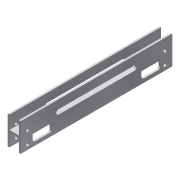
# Autodesk Inventor part: car frame
Saved by Autodesk Inventor 2015 (Build 190159000, 159)
## iProperties
Created: 2014-07-18
Part Number: car frame
Material: Generic
Document SubType Name: Modeling
Designer: Owner
Density: 1 g/cm^3
Appearance: Aluminum - Polished
Author: Owner
Autodesk Inventor part; units mm, degrees
ref_plane "YZ Plane" through (0, 0, 0) normal (1, 0, 0) x (0, 1, 0)
ref_plane "XZ Plane" through (0, 0, 0) normal (0, 1, 0) x (-1, 0, 0)
ref_plane "XY Plane" through (0, 0, 0) normal (0, 0, 1) x (1, 0, 0)
sketch "Sketch1" plane through (0, 0, 0) normal (0, 0, 1) x (1, 0, 0)
  line L0 (-6.35, 0) -> (6.35, 0)
  line L1 (-6.35, -2.3876) -> (6.35, -2.3876)
  line L2 (6.35, 0) -> (6.35, 17.8562)
  line L3 (6.35, 17.8562) -> (8.7376, 17.8562)
  line L4 (8.7376, 17.8562) -> (8.7376, -20.2438)
  line L5 (8.7376, -20.2438) -> (6.35, -20.2438)
  line L6 (6.35, -20.2438) -> (6.35, -2.3876)
  line L7 (-6.35, -2.3876) -> (-6.35, -20.2438)
  line L8 (-6.35, -20.2438) -> (-8.7376, -20.2438)
  line L9 (-8.7376, -20.2438) -> (-8.7376, 17.8562)
  line L10 (-8.7376, 17.8562) -> (-6.35, 17.8562)
  line L11 (-6.35, 17.8562) -> (-6.35, 0)
  point P0 (0, 0)
  point P1 (0, 0)
  dimension "d9" = 12.7
  dimension "d10" = 2.3876
  dimension "d11" = 17.8562
  dimension "d12" = 38.1
  dimension "d13" = 2.3876
  dimension "d14" = 2.3876
  dimension "d15" = 2.3876
  dimension "d16" = 17.8562
  dimension "d17" = 17.8562
  constraints: 24 end point, 7 parallel, 3 perpendicular, 2 collinear, 1 coincident, 1 horizontal, 1 midpoint
  measures "d9" distance of L0.start L0.end
  measures "d10" distance between parallel lines of L1 L0
  measures "d11" distance of L0.end L2.end
  measures "d12" distance of L3.end L4.end
  measures "d13" distance of L2.end L3.end
  measures "d14" distance of L4.end L5.end
  measures "d15" distance of L7.end L8.end
  measures "d16" distance of L10.end L0.start
  measures "d17" distance of L1.start L7.end
extrude "Extrusion1" add sketch "Sketch1" against normal blind 203.2
sketch "Sketch2" plane through (8.7376, -20.2438, 0) normal (1, 0, 0) x (0, 0, -1)
  point P0 (0, 0)
  point P1 (9.525, 6.35)
  dimension "d20" = 9.525
  dimension "d21" = 6.35
  measures "d20" horizontal distance of point (9.525, 6.35) point (0, 0)
  measures "d21" vertical distance of point (0, 0) point (9.525, 6.35)
hole "Hole1" at (8.7376, -13.8938, -9.525) direction (-1, 0, 0) diameter 4.2164 end through all
sketch "Sketch3" plane through (8.7376, -20.2438, 0) normal (1, 0, 0) x (0, 0, -1)
  point P0 (0, 38.1)
  point P1 (9.525, 23.0188)
  dimension "d29" = 15.0813
  dimension "d30" = 9.525
  measures "d29" vertical distance of point (0, 38.1) point (9.525, 23.019)
  measures "d30" horizontal distance of point (0, 38.1) point (9.525, 23.019)
hole "Hole2" at (8.7376, 2.775, -9.525) direction (-1, 0, 0) diameter 4.2164 end through all
sketch "Sketch4" plane through (8.7376, -20.2438, 0) normal (1, 0, 0) x (0, 0, -1)
  circle A0 centre (9.525, 23.0188) radius 2.1082 projected
  circle A1 centre (9.525, 6.35) radius 2.1082 projected
  line L0 (0, 0) -> (203.2, 0) projected
  line L1 (0, 38.1) -> (203.2, 38.1) projected
  line L2 (101.6, 38.1) -> (101.6, 0) construction
  circle A2 centre (193.675, 23.0188) radius 2.1082
  circle A3 centre (193.675, 6.35) radius 2.1082
  constraints: 2 centre point, 2 end point, 2 midpoint, 2 symmetric about line, 2 other
hole "Hole3" at (8.7376, 2.775, -193.675) at (8.7376, -13.8938, -193.675) direction (-1, 0, 0) diameter 4.2164 end through all
sketch "Sketch5" plane through (8.7376, -20.2438, 0) normal (1, 0, 0) x (0, 0, -1)
  line L0 (19.05, 5.08) -> (38.1, 5.08)
  line L1 (41.275, 8.255) -> (41.275, 14.605)
  line L2 (38.1, 17.78) -> (19.05, 17.78)
  line L3 (15.875, 14.605) -> (15.875, 8.255)
  arc A0 (19.05, 17.78) -> (15.875, 14.605) centre (19.05, 14.605) ccw
  arc A1 (41.275, 14.605) -> (38.1, 17.78) centre (38.1, 14.605) ccw
  arc A2 (38.1, 5.08) -> (41.275, 8.255) centre (38.1, 8.255) ccw
  arc A3 (15.875, 8.255) -> (19.05, 5.08) centre (19.05, 8.255) ccw
  point P0 (0, 0)
  point P1 (41.275, 17.78)
  point P2 (41.275, 5.08)
  point P3 (15.875, 17.78)
  point P4 (28.575, 17.78)
  point P5 (28.575, 17.78)
  dimension "d45" = 25.4
  dimension "d46" = 12.7
  dimension "d47" = 17.78
  dimension "d48" = 28.575
  dimension "d49" = 3.175
  constraints: 8 end point, 8 point on circle, 8 tangent, 6 point on line, 4 centre point, 3 equal radius, 2 parallel, 1 coincident, 1 horizontal, 1 midpoint, 1 perpendicular
  measures "d45" distance of point (15.875, 17.78) point (41.275, 17.78)
  measures "d46" distance of point (41.275, 17.78) point (41.275, 5.08)
  measures "d47" vertical distance of point (0, 0) point (28.575, 17.78)
  measures "d48" horizontal distance of point (0, 0) point (28.575, 17.78)
  measures "d49" radius of A0
extrude "Extrusion2" cut sketch "Sketch5" against normal through all
sketch "Sketch6" plane through (8.7376, -20.2438, 0) normal (1, 0, 0) x (0, 0, -1)
  arc A0 (19.05, 17.78) -> (15.875, 14.605) centre (19.05, 14.605) ccw projected
  arc A1 (41.275, 14.605) -> (38.1, 17.78) centre (38.1, 14.605) ccw projected
  arc A2 (38.1, 5.08) -> (41.275, 8.255) centre (38.1, 8.255) ccw projected
  arc A3 (15.875, 8.255) -> (19.05, 5.08) centre (19.05, 8.255) ccw projected
  line L0 (101.6, 38.1) -> (101.6, 0) construction
  arc A4 (187.325, 14.605) -> (184.15, 17.78) centre (184.15, 14.605) ccw
  line L1 (184.15, 17.78) -> (165.1, 17.78)
  arc A5 (165.1, 17.78) -> (161.925, 14.605) centre (165.1, 14.605) ccw
  line L2 (161.925, 14.605) -> (161.925, 8.255)
  arc A6 (161.925, 8.255) -> (165.1, 5.08) centre (165.1, 8.255) ccw
  line L3 (165.1, 5.08) -> (184.15, 5.08)
  arc A7 (184.15, 5.08) -> (187.325, 8.255) centre (184.15, 8.255) ccw
  line L4 (187.325, 8.255) -> (187.325, 14.605)
  constraints: 12 symmetric about line, 8 end point, 8 point on circle, 4 centre point, 4 other
extrude "Extrusion3" cut sketch "Sketch6" against normal through all
sketch "Sketch7" plane through (-6.35, 0, 0) normal (0, 1, 0) x (1, 0, 0)
  line L0 (15.0876, 19.05) -> (15.0876, 38.1) projected
  line L1 (-2.3876, 38.1) -> (-2.3876, 19.05) projected
  line L2 (-2.3876, 28.575) -> (15.0876, 28.575) construction
  line L3 (-2.3876, 28.575) -> (6.35, 28.575) construction
  dimension "d54" = 17.4752
  constraints: 4 end point, 3 midpoint
  measures "d54" distance of L2.start L2.end
hole "Hole4" at (0, 0, -28.575) direction (0, -1, 0) diameter 4.2164 end through all
sketch "Sketch8" plane through (-6.35, 0, 0) normal (0, 1, 0) x (1, 0, 0)
  circle A0 centre (6.35, 28.575) radius 2.1082 projected
  line L0 (0, 0) -> (0, 203.2) projected
  line L1 (15.0876, 101.6) -> (-2.2502, 101.6)
  circle A1 centre (6.35, 174.625) radius 2.1082
  constraints: 2 end point, 1 centre point, 1 perpendicular, 1 symmetric about line, 1 other
hole "Hole5" at (0, 0, -174.625) direction (0, -1, 0) diameter 4.2164 end through all
sketch "Sketch9" plane through (8.7376, -20.2438, 0) normal (1, 0, 0) x (0, 0, -1)
  line L0 (0, 20.2438) -> (203.2, 20.2438) projected
  line L1 (101.6, 38.1) -> (101.6, 0) construction
  line L2 (50.8, 20.2438) -> (152.4, 20.2438)
  line L3 (155.575, 23.4188) -> (155.575, 23.4188)
  line L4 (152.4, 26.5938) -> (50.8, 26.5938)
  line L5 (47.625, 23.4188) -> (47.625, 23.4188)
  arc A0 (50.8, 26.5938) -> (47.625, 23.4188) centre (50.8, 23.4188) ccw
  arc A1 (47.625, 23.4188) -> (50.8, 20.2438) centre (50.8, 23.4188) ccw
  arc A2 (155.575, 23.4188) -> (152.4, 26.5938) centre (152.4, 23.4188) ccw
  arc A3 (152.4, 20.2438) -> (155.575, 23.4188) centre (152.4, 23.4188) ccw
  point P0 (155.575, 26.5938)
  point P1 (155.575, 20.2438)
  point P2 (47.625, 26.5938)
  point P3 (101.6, 20.2438)
  dimension "d69" = 107.95
  dimension "d70" = 6.35
  dimension "d71" = 3.175
  constraints: 8 end point, 8 point on circle, 8 tangent, 6 point on line, 4 centre point, 3 equal radius, 2 midpoint, 2 parallel, 1 horizontal, 1 perpendicular
  measures "d69" distance of point (47.625, 26.594) point (155.575, 26.594)
  measures "d70" distance of point (155.575, 26.594) point (155.575, 20.244)
  measures "d71" radius of A0
extrude "Extrusion4" cut sketch "Sketch9" against normal through all
equation "\"d13\" = d10"
equation "\"d14\" = d10"
equation "\"d15\" = d10"
equation "\"d16\" = d11"
equation "\"d17\" = d11"
body "Solid1"
